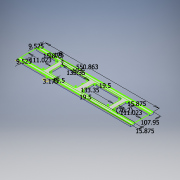
# Autodesk Inventor part: Drivetraintopbottom3
Saved by Autodesk Inventor 2017 (Build 210142000, 142)
## iProperties
Created: 2016-10-15
Part Number: Drivetraintopbottom3
Material: Aluminum 6061
Document SubType Name: Modeling
Designer: Kevin G
Density: 2.7 g/cm^3
Appearance: Aluminum - Flat
Author: Kevin G
Autodesk Inventor part; units mm, degrees
ref_plane "YZ Plane" through (0, 0, 0) normal (1, 0, 0) x (0, 1, 0)
ref_plane "XZ Plane" through (0, 0, 0) normal (0, 1, 0) x (-1, 0, 0)
ref_plane "XY Plane" through (0, 0, 0) normal (0, 0, 1) x (1, 0, 0)
ref_plane "Work Plane3" through (-147.218, 17.4273, 6.525) normal (0, 0, 1) x (1, 0, 0)
sketch "Sketch7" plane through (-147.218, 17.4273, 6.525) normal (0, 0, 1) x (1, 0, 0)
  line L0 (-4.0025, 142.0373) -> (8.6975, 142.0373)
  line L1 (8.6975, 166.8648) -> (534.16, 166.8648)
  line L2 (534.16, 151.8648) -> (546.86, 151.8648)
  line L3 (534.16, -35.9627) -> (546.86, -35.9627)
  line L4 (8.6975, 158.8648) -> (113.79, 158.8648)
  line L5 (113.79, 142.8648) -> (218.8825, 142.8648)
  line L6 (218.8825, 161.8648) -> (323.975, 161.8648)
  line L7 (323.975, 142.8648) -> (429.0675, 142.8648)
  circle A0 centre (117.7905, 87.3125) radius 3.175
  circle A1 centre (117.7905, -4.7625) radius 3.175
  circle A2 centre (12.6975, 87.3125) radius 3.175
  circle A3 centre (12.6975, -4.7625) radius 3.175
  circle A4 centre (222.8835, 87.3125) radius 3.175
  circle A5 centre (327.9765, 87.3125) radius 3.175
  circle A6 centre (433.0695, 87.3125) radius 3.175
  circle A7 centre (538.1625, 87.3125) radius 3.175
  circle A8 centre (222.8835, -4.7625) radius 3.175
  circle A9 centre (327.9765, -4.7625) radius 3.175
  circle A10 centre (433.0695, -4.7625) radius 3.175
  circle A11 centre (538.1625, -4.7625) radius 3.175
  line L8 (550.8625, -12.7) -> (550.8625, 3.175) projected
  line L9 (-0.0005, 95.25) -> (550.8625, 95.25)
  line L10 (550.8625, 95.25) -> (550.8625, -12.7)
  line L11 (550.8625, -12.7) -> (-0.0005, -12.7)
  line L12 (-0.0005, -12.7) -> (-0.0005, 95.25)
  line L13 (550.862, -9.525) -> (0, -9.525) projected
  point P0 (147.218, -17.4273)
  point P1 (431.29, 55.0373)
  dimension "d164" = 12.7
  dimension "d166" = 525.4625
  dimension "d167" = 12.7
  dimension "d168" = 105.0925
  dimension "d169" = 105.0925
  dimension "d170" = 105.0925
  dimension "d171" = 105.0925
  dimension "d172" = 105.0925
  dimension "d173" = 6.35
  dimension "d174" = 6.35
  dimension "d176" = 6.35
  dimension "d177" = 6.35
  dimension "d178" = 6.35
  dimension "d179" = 6.35
  dimension "d180" = 6.35
  dimension "d181" = 6.35
  dimension "d182" = 6.35
  dimension "d183" = 6.35
  dimension "d184" = 6.35
  dimension "d185" = 107.95
  dimension "d186" = 550.863
  dimension "d189" = 105.093
  dimension "d195" = 105.093
  dimension "d196" = 105.093
  dimension "d197" = 105.093
  dimension "d204" = 105.093
  dimension "d205" = 105.093
  dimension "d209" = 105.093
  dimension "d210" = 105.093
  dimension "d215" = 7.9375
  dimension "d217" = 7.9375
  dimension "d218" = 7.9375
  dimension "d219" = 7.9375
  dimension "d220" = 7.9375
  dimension "d221" = 7.9375
  dimension "d222" = 7.9375
  dimension "d223" = 105.093
  dimension "d224" = 105.093
  dimension "d225" = 7.9375
  dimension "d226" = 7.9375
  dimension "d227" = 7.9375
  dimension "d229" = 7.9375
  dimension "d231" = 12.7
  dimension "d232" = 12.7
  dimension "d233" = 12.698
  dimension "d234" = 7.9375
  dimension "d235" = 12.698
  constraints: 24 end point, 12 centre point, 9 horizontal, 2 parallel, 1 perpendicular
  measures "d164" distance of L0.start L0.end
  measures "d166" distance of L1.end L1.start
  measures "d167" distance of L3.start L3.end
  measures "d168" distance of L4.start L4.end
  measures "d169" distance of L5.start L5.end
  measures "d170" distance of L6.start L6.end
  measures "d171" distance of L7.end L7.start
  measures "d172" horizontal distance of L2.start L7.end
  measures "d173" diameter of A0
  measures "d174" diameter of A2
  measures "d176" diameter of A4
  measures "d177" diameter of A1
  measures "d178" diameter of A8
  measures "d179" diameter of A5
  measures "d180" diameter of A9
  measures "d181" diameter of A6
  measures "d182" diameter of A10
  measures "d183" diameter of A7
  measures "d184" diameter of A11
  measures "d185" distance of L9.end L8.start
  measures "d186" distance of L8.start L11.end
  measures "d189" distance of A0.centre A2.centre
  measures "d195" distance of A1.centre A3.centre
  measures "d196" distance of A4.centre A0.centre
  measures "d197" distance of A4.centre A5.centre
  measures "d204" distance of A6.centre A5.centre
  measures "d205" distance of A7.centre A6.centre
  measures "d209" distance of A10.centre A9.centre
  measures "d210" distance of A11.centre A10.centre
  measures "d215" distance from line of L11 A11.centre
  measures "d217" distance from line of L9 A4.centre
  measures "d218" distance from line of L9 A6.centre
  measures "d219" distance from line of A7.centre L9
  measures "d220" distance from line of L11 A10.centre
  measures "d221" distance from line of L11 A9.centre
  measures "d222" distance from line of L11 A8.centre
  measures "d223" distance of A9.centre A8.centre
  measures "d224" distance of A1.centre A8.centre
  measures "d225" distance from line of L11 A1.centre
  measures "d226" distance from line of L9 A0.centre
  measures "d227" distance from line of L9 A2.centre
  measures "d229" distance from line of L11 A3.centre
  measures "d231" distance from line of L10 A7.centre
  measures "d232" distance from line of L10 A11.centre
  measures "d233" distance from line of L12 A3.centre
  measures "d234" distance from line of L9 A5.centre
  measures "d235" distance from line of L12 A2.centre
hole "Hole5" [suppressed]
ref_plane "Work Plane4" through (0, 0, 9.525) normal (0, 0, 1) x (1, 0, 0)
sketch "Sketch8" plane through (0, 0, 9.525) normal (0, 0, 1) x (1, 0, 0)
  line L0 (292.6215, 88.8023) -> (292.6215, 28.6023)
  line L1 (273.1215, 85.1773) -> (273.1215, 32.2273)
  line L2 (-36.195, 28.6023) -> (-36.195, 88.8023)
  line L3 (-17.145, 85.1773) -> (-17.145, 32.2273)
  line L4 (-9.145, 24.2273) -> (108.205, 24.2273)
  line L5 (116.205, 32.2273) -> (116.205, 85.1773)
  line L6 (108.205, 93.1773) -> (-9.145, 93.1773)
  line L7 (147.772, 93.1773) -> (265.1215, 93.1773)
  line L8 (139.772, 85.1773) -> (139.772, 32.2273)
  line L9 (147.772, 24.2273) -> (265.1215, 24.2273)
  arc A0 (-9.145, 93.1773) -> (-17.145, 85.1773) centre (-9.145, 85.1773) ccw
  arc A1 (116.205, 85.1773) -> (108.205, 93.1773) centre (108.205, 85.1773) ccw
  arc A2 (-17.145, 32.2273) -> (-9.145, 24.2273) centre (-9.145, 32.2273) ccw
  arc A3 (108.205, 24.2273) -> (116.205, 32.2273) centre (108.205, 32.2273) ccw
  arc A4 (147.772, 93.1773) -> (139.772, 85.1773) centre (147.772, 85.1773) ccw
  arc A5 (273.1215, 85.1773) -> (265.1215, 93.1773) centre (265.1215, 85.1773) ccw
  arc A6 (265.1215, 24.2273) -> (273.1215, 32.2273) centre (265.1215, 32.2273) ccw
  arc A7 (139.772, 32.2273) -> (147.772, 24.2273) centre (147.772, 32.2273) ccw
  arc A8 (300.6215, 96.8023) -> (292.6215, 88.8023) centre (300.6215, 88.8023) ccw
  arc A9 (292.6215, 28.6023) -> (300.6215, 20.6023) centre (300.6215, 28.6023) ccw
  arc A10 (-36.195, 88.8023) -> (-44.195, 96.8023) centre (-44.195, 88.8023) ccw
  arc A11 (-44.195, 20.6023) -> (-36.195, 28.6023) centre (-44.195, 28.6023) ccw
  line L10 (-44.195, 96.8023) -> (-147.218, 96.8023)
  line L11 (-44.195, 20.6023) -> (-147.218, 20.6023)
  line L12 (300.6215, 96.8023) -> (403.6445, 96.8023)
  line L13 (300.6215, 20.6023) -> (403.6445, 20.6023)
  line L14 (-147.218, 112.6773) -> (403.6445, 112.6773)
  line L15 (403.6445, 112.6773) -> (403.6445, 4.7273)
  line L16 (403.6445, 4.7273) -> (-147.218, 4.7273)
  line L17 (-147.218, 4.7273) -> (-147.218, 112.6773)
  line L18 (-147.218, 109.5023) -> (403.6445, 109.5023)
  line L19 (-147.218, 99.9773) -> (403.6445, 99.9773)
  line L20 (-147.218, 7.9023) -> (403.6445, 7.9023)
  line L21 (-147.218, 17.4273) -> (403.6445, 17.4273)
  line L22 (292.6215, 88.8023) -> (292.6215, 28.6023)
  line L23 (273.1215, 85.1773) -> (273.1215, 32.2273)
  line L24 (-36.195, 28.6023) -> (-36.195, 88.8023)
  line L25 (-17.145, 85.1773) -> (-17.145, 32.2273)
  line L26 (-9.145, 24.2273) -> (108.205, 24.2273)
  line L27 (116.205, 32.2273) -> (116.205, 85.1773)
  line L28 (108.205, 93.1773) -> (-9.145, 93.1773)
  line L29 (147.772, 93.1773) -> (265.1215, 93.1773)
  line L30 (139.772, 85.1773) -> (139.772, 32.2273)
  line L31 (147.772, 24.2273) -> (265.1215, 24.2273)
  arc A12 (-9.145, 93.1773) -> (-17.145, 85.1773) centre (-9.145, 85.1773) ccw
  arc A13 (116.205, 85.1773) -> (108.205, 93.1773) centre (108.205, 85.1773) ccw
  arc A14 (-17.145, 32.2273) -> (-9.145, 24.2273) centre (-9.145, 32.2273) ccw
  arc A15 (108.205, 24.2273) -> (116.205, 32.2273) centre (108.205, 32.2273) ccw
  arc A16 (147.772, 93.1773) -> (139.772, 85.1773) centre (147.772, 85.1773) ccw
  arc A17 (273.1215, 85.1773) -> (265.1215, 93.1773) centre (265.1215, 85.1773) ccw
  arc A18 (265.1215, 24.2273) -> (273.1215, 32.2273) centre (265.1215, 32.2273) ccw
  arc A19 (139.772, 32.2273) -> (147.772, 24.2273) centre (147.772, 32.2273) ccw
  arc A20 (300.6215, 96.8023) -> (292.6215, 88.8023) centre (300.6215, 88.8023) ccw
  arc A21 (292.6215, 28.6023) -> (300.6215, 20.6023) centre (300.6215, 28.6023) ccw
  arc A22 (-36.195, 88.8023) -> (-44.195, 96.8023) centre (-44.195, 88.8023) ccw
  arc A23 (-44.195, 20.6023) -> (-36.195, 28.6023) centre (-44.195, 28.6023) ccw
  line L32 (-44.195, 96.8023) -> (-147.218, 96.8023)
  line L33 (-44.195, 20.6023) -> (-147.218, 20.6023)
  line L34 (300.6215, 96.8023) -> (403.6445, 96.8023)
  line L35 (300.6215, 20.6023) -> (403.6445, 20.6023)
  line L36 (-147.218, 112.6773) -> (403.6445, 112.6773)
  line L37 (403.6445, 112.6773) -> (403.6445, 4.7273)
  line L38 (403.6445, 4.7273) -> (-147.218, 4.7273)
  line L39 (-147.218, 4.7273) -> (-147.218, 112.6773)
  line L40 (-147.218, 109.5023) -> (403.6445, 109.5023)
  line L41 (-147.218, 99.9773) -> (403.6445, 99.9773)
  line L42 (-147.218, 7.9023) -> (403.6445, 7.9023)
  line L43 (-147.218, 17.4273) -> (403.6445, 17.4273)
  point P0 (0, 0)
  point P1 (0, 0)
  point P2 (116.205, 58.4523)
  point P3 (0, 0)
  point P4 (0, 0)
  point P5 (116.205, 58.4523)
  dimension "d250" = 133.35
  dimension "d251" = 133.3495
  dimension "d252" = 8
  dimension "d253" = 550.8625
  dimension "d254" = 107.95
  dimension "d255" = 111.023
  dimension "d256" = 111.023
  dimension "d257" = 19.5
  dimension "d258" = 19.5
  dimension "d259" = 19.5
  dimension "d260" = 19.5
  dimension "d261" = 15.875
  dimension "d262" = 3.175
  dimension "d263" = 9.525
  dimension "d264" = 3.175
  dimension "d265" = 9.525
  dimension "d266" = 15.875
  dimension "d267" = 15.875
  dimension "d268" = 76.2
  dimension "d269" = 133.35
  dimension "d270" = 133.3495
  dimension "d271" = 8
  dimension "d272" = 550.8625
  dimension "d273" = 107.95
  dimension "d274" = 111.023
  dimension "d275" = 111.023
  dimension "d276" = 19.5
  dimension "d277" = 19.5
  dimension "d278" = 19.5
  dimension "d279" = 19.5
  dimension "d280" = 15.875
  dimension "d281" = 3.175
  dimension "d282" = 9.525
  dimension "d283" = 3.175
  dimension "d284" = 9.525
  dimension "d285" = 15.875
  dimension "d286" = 15.875
  dimension "d287" = 76.2
  constraints: 88 end point, 48 point on circle, 40 tangent, 26 point on line, 24 centre point, 22 equal radius, 10 perpendicular, 8 horizontal, 8 parallel, 6 vertical
  measures "d250" distance between parallel lines of L5 L3
  measures "d251" distance between parallel lines of L1 L8
  measures "d252" radius of A0
  measures "d253" distance of L14.start L14.end
  measures "d254" distance of L14.end L15.end
  measures "d255" distance between parallel lines of L2 L17
  measures "d256" distance between parallel lines of L15 L0
  measures "d257" distance between parallel lines of L14 L6
  measures "d258" distance between parallel lines of L16 L4
  measures "d259" distance between parallel lines of L14 L7
  measures "d260" distance between parallel lines of L16 L9
  measures "d261" distance between parallel lines of L14 L10
  measures "d262" distance between parallel lines of L14 L18
  measures "d263" distance between parallel lines of L18 L19
  measures "d264" distance between parallel lines of L20 L16
  measures "d265" distance between parallel lines of L21 L20
  measures "d266" distance between parallel lines of L14 L12
  measures "d267" distance between parallel lines of L16 L13
  measures "d268" distance between parallel lines of L13 L12
  measures "d269" distance between parallel lines of L27 L25
  measures "d270" distance between parallel lines of L23 L30
  measures "d271" radius of A12
  measures "d272" distance of L36.start L36.end
  measures "d273" distance of L36.end L37.end
  measures "d274" distance between parallel lines of L24 L39
  measures "d275" distance between parallel lines of L37 L22
  measures "d276" distance between parallel lines of L36 L28
  measures "d277" distance between parallel lines of L38 L26
  measures "d278" distance between parallel lines of L36 L29
  measures "d279" distance between parallel lines of L38 L31
  measures "d280" distance between parallel lines of L36 L32
  measures "d281" distance between parallel lines of L36 L40
  measures "d282" distance between parallel lines of L40 L41
  measures "d283" distance between parallel lines of L42 L38
  measures "d284" distance between parallel lines of L43 L42
  measures "d285" distance between parallel lines of L36 L34
  measures "d286" distance between parallel lines of L38 L35
  measures "d287" distance between parallel lines of L35 L34
extrude "Extrusion4" add sketch "Sketch8" along normal blind 9.525 contours L0 A9 L13 L15 L21 L17 L11 A11 L2 A10 L10 L19 L12 A8 | L19 L17 L18 L15 | L15 L20 L17 L21 | L18 L17 L14 L15 | L15 L16 L17 L20
sketch "Sketch9" plane through (0, 0, 19.05) normal (0, 0, 1) x (1, 0, 0)
  line L0 (292.6215, 88.8023) -> (292.6215, 28.6023)
  line L1 (273.1215, 85.1773) -> (273.1215, 32.2273)
  line L2 (-36.195, 28.6023) -> (-36.195, 88.8023)
  line L3 (-17.145, 85.1773) -> (-17.145, 32.2273)
  line L4 (-9.145, 24.2273) -> (108.205, 24.2273)
  line L5 (116.205, 32.2273) -> (116.205, 85.1773)
  line L6 (108.205, 93.1773) -> (-9.145, 93.1773)
  line L7 (147.772, 93.1773) -> (265.1215, 93.1773)
  line L8 (139.772, 85.1773) -> (139.772, 32.2273)
  line L9 (147.772, 24.2273) -> (265.1215, 24.2273)
  arc A0 (-9.145, 93.1773) -> (-17.145, 85.1773) centre (-9.145, 85.1773) ccw
  arc A1 (116.205, 85.1773) -> (108.205, 93.1773) centre (108.205, 85.1773) ccw
  arc A2 (-17.145, 32.2273) -> (-9.145, 24.2273) centre (-9.145, 32.2273) ccw
  arc A3 (108.205, 24.2273) -> (116.205, 32.2273) centre (108.205, 32.2273) ccw
  arc A4 (147.772, 93.1773) -> (139.772, 85.1773) centre (147.772, 85.1773) ccw
  arc A5 (273.1215, 85.1773) -> (265.1215, 93.1773) centre (265.1215, 85.1773) ccw
  arc A6 (265.1215, 24.2273) -> (273.1215, 32.2273) centre (265.1215, 32.2273) ccw
  arc A7 (139.772, 32.2273) -> (147.772, 24.2273) centre (147.772, 32.2273) ccw
  arc A8 (300.6215, 96.8023) -> (292.6215, 88.8023) centre (300.6215, 88.8023) ccw
  arc A9 (292.6215, 28.6023) -> (300.6215, 20.6023) centre (300.6215, 28.6023) ccw
  arc A10 (-36.195, 88.8023) -> (-44.195, 96.8023) centre (-44.195, 88.8023) ccw
  arc A11 (-44.195, 20.6023) -> (-36.195, 28.6023) centre (-44.195, 28.6023) ccw
  line L10 (-44.195, 96.8023) -> (-147.218, 96.8023)
  line L11 (-44.195, 20.6023) -> (-147.218, 20.6023)
  line L12 (300.6215, 96.8023) -> (403.6445, 96.8023)
  line L13 (300.6215, 20.6023) -> (403.6445, 20.6023)
  line L14 (-147.218, 112.6773) -> (403.6445, 112.6773)
  line L15 (403.6445, 112.6773) -> (403.6445, 4.7273)
  line L16 (403.6445, 4.7273) -> (-147.218, 4.7273)
  line L17 (-147.218, 4.7273) -> (-147.218, 112.6773)
  line L18 (-147.218, 109.5023) -> (403.6445, 109.5023)
  line L19 (-147.218, 99.9773) -> (403.6445, 99.9773)
  line L20 (-147.218, 7.9023) -> (403.6445, 7.9023)
  line L21 (-147.218, 17.4273) -> (403.6445, 17.4273)
  line L22 (292.6215, 88.8023) -> (292.6215, 28.6023)
  line L23 (273.1215, 85.1773) -> (273.1215, 32.2273)
  line L24 (-36.195, 28.6023) -> (-36.195, 88.8023)
  line L25 (-17.145, 85.1773) -> (-17.145, 32.2273)
  line L26 (-9.145, 24.2273) -> (108.205, 24.2273)
  line L27 (116.205, 32.2273) -> (116.205, 85.1773)
  line L28 (108.205, 93.1773) -> (-9.145, 93.1773)
  line L29 (147.772, 93.1773) -> (265.1215, 93.1773)
  line L30 (139.772, 85.1773) -> (139.772, 32.2273)
  line L31 (147.772, 24.2273) -> (265.1215, 24.2273)
  arc A12 (-9.145, 93.1773) -> (-17.145, 85.1773) centre (-9.145, 85.1773) ccw
  arc A13 (116.205, 85.1773) -> (108.205, 93.1773) centre (108.205, 85.1773) ccw
  arc A14 (-17.145, 32.2273) -> (-9.145, 24.2273) centre (-9.145, 32.2273) ccw
  arc A15 (108.205, 24.2273) -> (116.205, 32.2273) centre (108.205, 32.2273) ccw
  arc A16 (147.772, 93.1773) -> (139.772, 85.1773) centre (147.772, 85.1773) ccw
  arc A17 (273.1215, 85.1773) -> (265.1215, 93.1773) centre (265.1215, 85.1773) ccw
  arc A18 (265.1215, 24.2273) -> (273.1215, 32.2273) centre (265.1215, 32.2273) ccw
  arc A19 (139.772, 32.2273) -> (147.772, 24.2273) centre (147.772, 32.2273) ccw
  arc A20 (300.6215, 96.8023) -> (292.6215, 88.8023) centre (300.6215, 88.8023) ccw
  arc A21 (292.6215, 28.6023) -> (300.6215, 20.6023) centre (300.6215, 28.6023) ccw
  arc A22 (-36.195, 88.8023) -> (-44.195, 96.8023) centre (-44.195, 88.8023) ccw
  arc A23 (-44.195, 20.6023) -> (-36.195, 28.6023) centre (-44.195, 28.6023) ccw
  line L32 (-44.195, 96.8023) -> (-147.218, 96.8023)
  line L33 (-44.195, 20.6023) -> (-147.218, 20.6023)
  line L34 (300.6215, 96.8023) -> (403.6445, 96.8023)
  line L35 (300.6215, 20.6023) -> (403.6445, 20.6023)
  line L36 (-147.218, 112.6773) -> (403.6445, 112.6773)
  line L37 (403.6445, 112.6773) -> (403.6445, 4.7273)
  line L38 (403.6445, 4.7273) -> (-147.218, 4.7273)
  line L39 (-147.218, 4.7273) -> (-147.218, 112.6773)
  line L40 (-147.218, 109.5023) -> (403.6445, 109.5023)
  line L41 (-147.218, 99.9773) -> (403.6445, 99.9773)
  line L42 (-147.218, 7.9023) -> (403.6445, 7.9023)
  line L43 (-147.218, 17.4273) -> (403.6445, 17.4273)
  point P0 (0, 0)
  point P1 (0, 0)
  point P2 (0, 0)
  point P3 (116.205, 58.4523)
  point P4 (0, 0)
  point P5 (0, 0)
  point P6 (116.205, 58.4523)
  dimension "d290" = 133.35
  dimension "d291" = 133.3495
  dimension "d292" = 8
  dimension "d293" = 550.8625
  dimension "d294" = 107.95
  dimension "d295" = 111.023
  dimension "d296" = 111.023
  dimension "d297" = 19.5
  dimension "d298" = 19.5
  dimension "d299" = 19.5
  dimension "d300" = 19.5
  dimension "d301" = 15.875
  dimension "d302" = 3.175
  dimension "d303" = 9.525
  dimension "d304" = 3.175
  dimension "d305" = 9.525
  dimension "d306" = 15.875
  dimension "d307" = 15.875
  dimension "d308" = 76.2
  dimension "d309" = 133.35
  dimension "d310" = 133.3495
  dimension "d311" = 8
  dimension "d312" = 550.8625
  dimension "d313" = 107.95
  dimension "d314" = 111.023
  dimension "d315" = 111.023
  dimension "d316" = 19.5
  dimension "d317" = 19.5
  dimension "d318" = 19.5
  dimension "d319" = 19.5
  dimension "d320" = 15.875
  dimension "d321" = 3.175
  dimension "d322" = 9.525
  dimension "d323" = 3.175
  dimension "d324" = 9.525
  dimension "d325" = 15.875
  dimension "d326" = 15.875
  dimension "d327" = 76.2
  constraints: 88 end point, 48 point on circle, 40 tangent, 26 point on line, 24 centre point, 22 equal radius, 10 perpendicular, 8 horizontal, 8 parallel, 6 vertical
  measures "d290" distance between parallel lines of L5 L3
  measures "d291" distance between parallel lines of L1 L8
  measures "d292" radius of A0
  measures "d293" distance of L14.start L14.end
  measures "d294" distance of L14.end L15.end
  measures "d295" distance between parallel lines of L2 L17
  measures "d296" distance between parallel lines of L15 L0
  measures "d297" distance between parallel lines of L14 L6
  measures "d298" distance between parallel lines of L16 L4
  measures "d299" distance between parallel lines of L14 L7
  measures "d300" distance between parallel lines of L16 L9
  measures "d301" distance between parallel lines of L14 L10
  measures "d302" distance between parallel lines of L14 L18
  measures "d303" distance between parallel lines of L18 L19
  measures "d304" distance between parallel lines of L20 L16
  measures "d305" distance between parallel lines of L21 L20
  measures "d306" distance between parallel lines of L14 L12
  measures "d307" distance between parallel lines of L16 L13
  measures "d308" distance between parallel lines of L13 L12
  measures "d309" distance between parallel lines of L27 L25
  measures "d310" distance between parallel lines of L23 L30
  measures "d311" radius of A12
  measures "d312" distance of L36.start L36.end
  measures "d313" distance of L36.end L37.end
  measures "d314" distance between parallel lines of L24 L39
  measures "d315" distance between parallel lines of L37 L22
  measures "d316" distance between parallel lines of L36 L28
  measures "d317" distance between parallel lines of L38 L26
  measures "d318" distance between parallel lines of L36 L29
  measures "d319" distance between parallel lines of L38 L31
  measures "d320" distance between parallel lines of L36 L32
  measures "d321" distance between parallel lines of L36 L40
  measures "d322" distance between parallel lines of L40 L41
  measures "d323" distance between parallel lines of L42 L38
  measures "d324" distance between parallel lines of L43 L42
  measures "d325" distance between parallel lines of L36 L34
  measures "d326" distance between parallel lines of L38 L35
  measures "d327" distance between parallel lines of L35 L34
body "Solid2"
